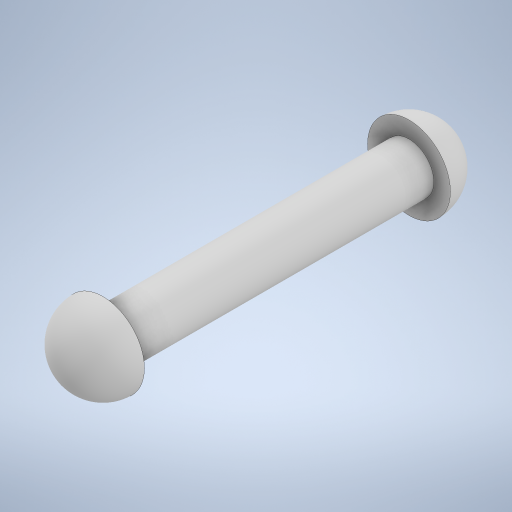
# Autodesk Inventor part: atividade_14A_pino37
Saved by Autodesk Inventor 2024.2 (Build 282272000, 272)
## iProperties
Created: 2024-03-04
Part Number: atividade_14A_pino37
Material: Generic
Document SubType Name: Modeling
Designer: 082220042
Density: 1 g/cm^3
Appearance: Default
Author: 082220042
Autodesk Inventor part; units mm, degrees
ref_plane "YZ Plane" through (0, 0, 0) normal (1, 0, 0) x (0, 1, 0)
ref_plane "XZ Plane" through (0, 0, 0) normal (0, 1, 0) x (-1, 0, 0)
ref_plane "XY Plane" through (0, 0, 0) normal (0, 0, 1) x (1, 0, 0)
sketch "Sketch1" plane through (0, 0, 0) normal (1, 0, 0) x (0, 1, 0)
  line L0 (0, 0) -> (0, 0)
  line L1 (0, 0) -> (0, 0) construction
  line L2 (5, -5) -> (5, -5)
  line L3 (5, -5) -> (3, -5)
  line L4 (3, -5) -> (3, -42)
  line L5 (3, -42) -> (5, -42)
  line L6 (5, -42) -> (5, -42)
  line L7 (0, -47) -> (0, -47)
  line L8 (0, -47) -> (0, 0)
  arc A0 (5, -5) -> (0, 0) centre (0, -5) ccw
  arc A1 (0, -47) -> (5, -42) centre (0, -42) ccw
  point P0 (5, 0)
  point P1 (5, -47)
  dimension "d4" = 5
  dimension "d5" = 0
  dimension "d6" = 5
  dimension "d7" = 2
  dimension "d8" = 37
  dimension "d9" = 90
  dimension "d10" = 2
  dimension "d11" = 5
  dimension "d12" = 5
  dimension "d13" = 5
  constraints: 18 end point, 6 point on line, 5 perpendicular, 4 point on circle, 4 tangent, 2 centre point, 2 horizontal, 1 collinear
  measures "d4" distance of L0.start point (5, 0)
  measures "d5" distance between parallel lines of L0 L1
  measures "d6" distance of point (5, 0) L2.end
  measures "d7" distance of L2.end L3.end
  measures "d8" distance of L3.end L4.end
  measures "d9" angle of L4 L3
  measures "d10" distance of L4.end L5.end
  measures "d11" distance of L5.end point (5, -47)
  measures "d12" radius of A0
  measures "d13" radius of A1
revolve "Revolution1" add sketch "Sketch1" angle 360 about axis through (0, 0, -47) along (0, 0, 1)
body "Solid1"
